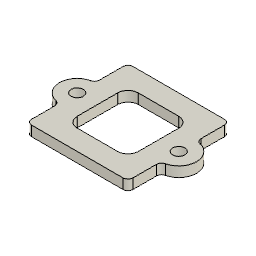
ELP Camera Lens Spacer (Autodesk Fusion 360 design; units mm, degrees)
Autodesk Fusion 360 part; units mm, degrees
note: some values were not read from the file. Set by a fixed rule: which sketch regions a step uses.
sketch "Sketch1" plane through (0, 0, 0) normal (0, 0, 1) x (1, 0, 0)
  line L0 (4, 6) -> (-4, 6)
  line L1 (-6, 4) -> (-6, -4)
  line L2 (-4, -6) -> (4, -6)
  line L3 (6, -4) -> (6, 4)
  line L4 (6, 6) -> (-6, -6) construction
  line L5 (-6, 6) -> (6, -6) construction
  line L6 (9, -10) -> (-9, -10)
  line L7 (-10, -9) -> (-10, 9)
  line L8 (-9, 10) -> (9, 10)
  line L9 (10, 9) -> (10, -9)
  line L10 (10, -10) -> (-10, 10) construction
  line L11 (-10, -10) -> (10, 10) construction
  circle A0 centre (10, 0) radius 1.2
  circle A1 centre (-10, 0) radius 1.2
  circle A2 centre (10, 0) radius 3.5
  circle A3 centre (-10, 0) radius 3.5
  arc A4 (-9, 10) -> (-10, 9) centre (-9, 9) ccw
  arc A5 (10, 9) -> (9, 10) centre (9, 9) ccw
  arc A6 (-10, -9) -> (-9, -10) centre (-9, -9) ccw
  arc A7 (9, -10) -> (10, -9) centre (9, -9) ccw
  arc A8 (-4, 6) -> (-6, 4) centre (-4, 4) ccw
  arc A9 (6, 4) -> (4, 6) centre (4, 4) ccw
  arc A10 (-6, -4) -> (-4, -6) centre (-4, -4) ccw
  arc A11 (4, -6) -> (6, -4) centre (4, -4) ccw
  dimension "d1" = 12
  dimension "d2" = 12
  dimension "d3" = 20
  dimension "d4" = 20
  dimension "d5" = 2.4
  dimension "d6" = 2.4
  dimension "d7" = 7
  dimension "d8" = 7
  dimension "d9" = 10
  dimension "d10" = 10
  dimension "d11" = 1
  dimension "d12" = 1
  dimension "d13" = 1
  dimension "d14" = 2
  dimension "d15" = 2
  dimension "d16" = 2
  dimension "d17" = 2
  constraint horizontal L0
  constraint perpendicular L0 L1
  constraint parallel L0 L2
  constraint parallel L1 L3
  constraint coincident L4 origin
  constraint coincident L5 origin
  constraint horizontal L6
  constraint perpendicular L6 L7
  constraint parallel L6 L8
  constraint parallel L7 L9
  constraint coincident L10 origin
  constraint coincident L11 origin
  constraint concentric A0 A2
  constraint concentric A1 A3
  constraint coincident L10.end L7
  constraint coincident L10.end L8
  constraint tangent L7 A4
  constraint tangent L8 A4
  constraint coincident L11.end L8
  constraint coincident L11.end L9
  constraint tangent L8 A5
  constraint tangent L9 A5
  constraint equal A4 A5
  constraint coincident L11.start L7
  constraint coincident L11.start L6
  constraint tangent L7 A6
  constraint tangent L6 A6
  constraint coincident L10.start L6
  constraint coincident L10.start L9
  constraint tangent L6 A7
  constraint tangent L9 A7
  constraint coincident L5.start L1
  constraint coincident L5.start L0
  constraint tangent L1 A8
  constraint tangent L0 A8
  constraint coincident L4.start L0
  constraint coincident L4.start L3
  constraint tangent L0 A9
  constraint tangent L3 A9
  constraint coincident L4.end L1
  constraint coincident L4.end L2
  constraint tangent L1 A10
  constraint tangent L2 A10
  constraint coincident L5.end L2
  constraint coincident L5.end L3
  constraint tangent L2 A11
  constraint tangent L3 A11
  measures "d1" distance of L4.end L5.end
  measures "d2" distance of L5.start L4.end
  measures "d3" distance of L10.end L11.end
  measures "d4" distance of L11.start L10.end
  measures "d5" diameter of A0
  measures "d6" diameter of A1
  measures "d7" diameter of A2
  measures "d8" diameter of A3
  measures "d9" distance of origin A0.centre
  measures "d10" distance of origin A1.centre
  measures "d11" radius of A4
  measures "d12" radius of A6
  measures "d13" radius of A7
  measures "d14" radius of A8
  measures "d15" radius of A9
  measures "d16" radius of A10
  measures "d17" radius of A11
extrude "Extrude1" add sketch "Sketch1" along normal blind 2 contours L6 L7 L8 L9 A2 A3 A4 A5 A6 A7 | L9 A0 A2 | L9 A0 A2 | L7 A1 A3 | L7 A1 A3
fillet "Fillet1" radius 1 4 edges at (10, -3.5, 1) (10, 3.5, 1) (-10, 3.5, 1) (-10, -3.5, 1)
